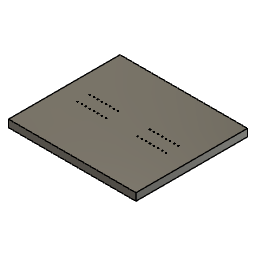
Soldering Fixture v1 (Autodesk Fusion 360 design; units mm, degrees)
Autodesk Fusion 360 part; units mm, degrees
sketch "Sketch1" plane through (0, 0, 0) normal (0, 1, 0) x (1, 0, 0)
  line L0 (0, 0) -> (80, 0)
  line L1 (80, 0) -> (80, 70)
  line L2 (80, 70) -> (0, 70)
  line L3 (0, 70) -> (0, 0)
  dimension "d1" = 80
  dimension "d2" = 70
  constraint horizontal L0
  constraint vertical L1
  constraint horizontal L2
  constraint vertical L3
  constraint coincident L0.start L3.end
  measures "d1" distance of L0.start L0.end
  measures "d2" distance of L0.start L2.end
extrude "Extrude1" add sketch "Sketch1" along normal blind 4.6
sketch "Sketch2" plane through (0, 4.6, 0) normal (0, 1, 0) x (-1, 0, 0)
  line L0 (0, -70) -> (0, 0)
  line L1 (0, 0) -> (-80, 0)
  line L2 (-80, 0) -> (-80, -70)
  line L3 (-80, -70) -> (0, -70)
  line L4 (0, -38.81) -> (-80, -38.81) construction
  line L5 (0, -31.19) -> (-80, -31.19) construction
  line L6 (-30, -38.81) -> (-30, -31.19) construction
  line L7 (-50, -38.81) -> (-50, -31.19) construction
  point P0 (-30, -38.81)
  point P1 (-30, -31.19)
  point P2 (-27.46, -38.81)
  point P3 (-27.46, -31.19)
  point P4 (-24.92, -38.81)
  point P5 (-24.92, -31.19)
  point P6 (-22.38, -38.81)
  point P7 (-22.38, -31.19)
  point P8 (-19.84, -38.81)
  point P9 (-19.84, -31.19)
  point P10 (-17.3, -38.81)
  point P11 (-17.3, -31.19)
  point P12 (-14.76, -38.81)
  point P13 (-14.76, -31.19)
  point P14 (-12.22, -38.81)
  point P15 (-12.22, -31.19)
  point P16 (-50, -38.81)
  point P17 (-50, -31.19)
  point P18 (-52.54, -38.81)
  point P19 (-52.54, -31.19)
  point P20 (-55.08, -38.81)
  point P21 (-55.08, -31.19)
  point P22 (-57.62, -38.81)
  point P23 (-57.62, -31.19)
  point P24 (-60.16, -38.81)
  point P25 (-60.16, -31.19)
  point P26 (-62.7, -38.81)
  point P27 (-62.7, -31.19)
  point P28 (-65.24, -38.81)
  point P29 (-65.24, -31.19)
  point P30 (-67.78, -38.81)
  point P31 (-67.78, -31.19)
  dimension "d9" = 2.54
  dimension "d10" = 0
  dimension "d13" = -2.54
  dimension "d14" = 0
  constraint coincident L0 L4.start
  constraint coincident L2 L4.end
  constraint coincident L0 L5.start
  constraint coincident L2 L5.end
  constraint coincident L4 P0
  constraint coincident L5 P1
  constraint perpendicular L5 L6
  constraint coincident L4 P16
  constraint coincident L5 P17
  constraint coincident P0 L6.start
  constraint coincident P1 L6.end
  constraint coincident P16 L7.start
  constraint coincident P17 L7.end
hole "Hole1" at (17.3, 4.6, -38.81) at (17.3, 4.6, -31.19) at (55.08, 4.6, -38.81) at (14.76, 4.6, -38.81) at (60.16, 4.6, -31.19) at (50, 4.6, -38.81) at (57.62, 4.6, -31.19) at (22.38, 4.6, -31.19) at (67.78, 4.6, -31.19) at (52.54, 4.6, -31.19) at (65.24, 4.6, -31.19) at (27.46, 4.6, -38.81) at (57.62, 4.6, -38.81) at (30, 4.6, -31.19) at (24.92, 4.6, -38.81) at (14.76, 4.6, -31.19) at (19.84, 4.6, -38.81) at (12.22, 4.6, -31.19) at (50, 4.6, -31.19) at (30, 4.6, -31.19) at (60.16, 4.6, -38.81) at (62.7, 4.6, -38.81) at (30, 4.6, -38.81) at (67.78, 4.6, -38.81) at (27.46, 4.6, -31.19) at (22.38, 4.6, -38.81) at (62.7, 4.6, -31.19) at (50, 4.6, -38.81) at (55.08, 4.6, -31.19) at (65.24, 4.6, -38.81) at (52.54, 4.6, -38.81) at (50, 4.6, -31.19) at (19.84, 4.6, -31.19) at (24.92, 4.6, -31.19) at (30, 4.6, -38.81) at (12.22, 4.6, -38.81) direction (0, -1, 0) diameter 0.8128 end through all
